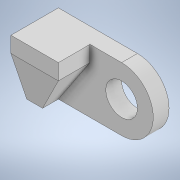
# Autodesk Inventor part: 件27
Saved by Autodesk Inventor 2020 (Build 240168000, 168)
## iProperties
Created: 2020-10-30
Part Number: 件27
Material: 一般
Document SubType Name: Modeling
Designer: USER
Density: 1 g/cm^3
Appearance: 預設
Author: USER
Autodesk Inventor part; units mm, degrees
ref_plane "YZ Plane" through (0, 0, 0) normal (1, 0, 0) x (0, 1, 0)
ref_plane "XZ Plane" through (0, 0, 0) normal (0, 1, 0) x (-1, 0, 0)
ref_plane "XY Plane" through (0, 0, 0) normal (0, 0, 1) x (1, 0, 0)
sketch "草圖1" plane through (0, 0, 0) normal (0, 0, 1) x (1, 0, 0)
  line L0 (15, -20) -> (-35, -20)
  line L1 (-35, -20) -> (-35, 20)
  line L2 (-35, 20) -> (15, 20)
  line L3 (35, 0) -> (35, 0)
  line L4 (35, -20) -> (-35, 20) construction
  line L5 (-35, -20) -> (35, 20) construction
  circle A0 centre (15, 0) radius 10
  arc A1 (35, 0) -> (15, 20) centre (15, 0) ccw
  arc A2 (15, -20) -> (35, 0) centre (15, 0) ccw
  point P0 (0, 0)
  dimension "d0" = 70
  dimension "d1" = 40
  dimension "d2" = 20
  dimension "d3" = 20
  dimension "d4" = 20
  dimension "d5" = 20
  constraints: 12 end point, 4 point on circle, 4 point on line, 4 tangent, 3 centre point, 2 midpoint, 2 parallel, 1 concentric, 1 horizontal, 1 perpendicular
  measures "d0" distance between parallel lines of L3 L1
  measures "d1" distance between parallel lines of L0 L2
  measures "d2" distance from line of L0 A0.centre
  measures "d3" distance from line of L3 A0.centre
  measures "d4" diameter of A0
  measures "d5" radius of A1
extrude "擠出1" add sketch "草圖1" along normal blind 10
sketch "草圖2" plane through (0, 0, 10) normal (0, 0, 1) x (1, 0, 0)
  line L0 (15, 20) -> (-35, 20) projected
  line L1 (-35, 20) -> (-5, 20)
  line L2 (-5, 20) -> (-5, 10)
  line L3 (-5, 10) -> (-35, 10)
  line L4 (-35, 10) -> (-35, 20)
  point P0 (0, 0)
  dimension "d8" = 10
  dimension "d9" = 30
  constraints: 8 end point, 2 parallel, 1 horizontal, 1 perpendicular
  measures "d8" distance between parallel lines of L3 L0
  measures "d9" distance between parallel lines of L2 L4
extrude "擠出2" add sketch "草圖2" along normal blind 20
sketch "草圖4" plane through (-35, -20, 0) normal (0, -1, 0) x (1, 0, 0)
  line L0 (0, 10) -> (50, 10) projected
  line L1 (0, 10) -> (10, 10)
  line L2 (10, 10) -> (10, 20)
  line L3 (10, 20) -> (0, 20)
  line L4 (0, 20) -> (0, 10)
  point P0 (35, 0)
  dimension "d12" = 10
  dimension "d13" = 10
  constraints: 8 end point, 2 parallel, 1 horizontal, 1 perpendicular
  measures "d12" distance between parallel lines of L0 L3
  measures "d13" distance between parallel lines of L2 L4
loft "斷面混成1" add profiles "草圖4" section 2 edges at (-20, 10, 10) (-5, 10, 20) (-20, 10, 30) (-35, 10, 20)
